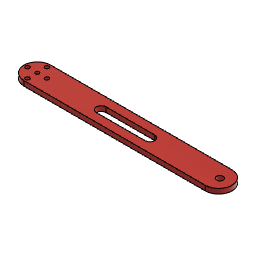
pendulum (Autodesk Fusion 360 design; units mm, degrees)
Autodesk Fusion 360 part; units mm, degrees
sketch "Sketch1" plane through (0, 0, 0) normal (0, 1, 0) x (1, 0, 0)
  line L0 (-90.5, 11) -> (80.5, 11)
  line L1 (80.5, 11) -> (80.5, -11)
  line L2 (80.5, -11) -> (-90.5, -11)
  line L3 (-90.5, -11) -> (-90.5, 11)
  circle A0 centre (-71.5, 0) radius 1.65
  circle A1 centre (-79.5, 8) radius 1.65
  circle A2 centre (-87.5, 0) radius 1.65
  circle A3 centre (-79.5, -8) radius 1.65
  circle A4 centre (70.5, 0) radius 2.75
  point P0 (-79.5, 0)
  dimension "d6" = 11
  dimension "d7" = 22
  dimension "d10" = 3.3
  dimension "d11" = 8
  dimension "d13" = 360
  dimension "d14" = 5.5
  dimension "d15" = 10
  dimension "d16" = 150
  dimension "d17" = 11
  dimension "d18" = 11
  dimension "d19" = 11
  constraint horizontal L0
  constraint vertical L1
  constraint horizontal L2
  constraint vertical L3
  measures "d6" distance of origin L2
  measures "d7" distance of L0.start L2.end
  measures "d10" diameter of A0
  measures "d11" distance of P0 A0.centre
  measures "d14" diameter of A4
  measures "d15" distance of L1 A4.centre
  measures "d16" distance of P0 A4.centre
  measures "d17" distance of L0 A4.centre
  measures "d18" distance of L0 P0
  measures "d19" distance of L3 P0
extrude "Extrude1" add sketch "Sketch1" along normal blind 4
fillet "Fillet1" radius 11 2 edges at (80.5, 2, -11) (80.5, 2, 11)
fillet "Fillet2" radius 11 2 edges at (-90.5, 2, 11) (-90.5, 2, -11)
sketch "Sketch3" plane through (0, 4, 0) normal (0, 1, 0) x (-1, 0, 0)
  circle A0 centre (79.5, -8) radius 1.65
  circle A1 centre (87.5, 0) radius 1.65
  circle A2 centre (79.5, 8) radius 1.65
  circle A3 centre (-70.5, 0) radius 2.75
  circle A4 centre (71.5, 0) radius 1.65
  arc A5 (79.5, -11) -> (79.5, 11) centre (79.5, 0) ccw
  line L0 (79.5, 11) -> (-69.5, 11)
  arc A6 (-69.5, 11) -> (-69.5, -11) centre (-69.5, 0) ccw
  line L1 (-69.5, -11) -> (79.5, -11)
  line L2 (27, 4) -> (-13, 4)
  arc A7 (-13, 4) -> (-13, -4) centre (-13, 0) ccw
  line L3 (-13, -4) -> (27, -4)
  arc A8 (27, -4) -> (27, 4) centre (27, 0) ccw
  line L4 (27, 0) -> (-13, 0) construction
  dimension "d24" = 8
  dimension "d30" = 40
  constraint tangent L2 A7
  constraint tangent A7 L3
  constraint parallel L2 L3
  constraint tangent L3 A8
  constraint tangent L2 A8
  constraint parallel L1 L4
  measures "d24" diameter of A7
  measures "d30" distance of A8.centre A7.centre
extrude "Extrude2" cut sketch "Sketch3" against normal up to surface (4 mm away) contours L2 A7 L3 A8
sketch "Sketch4" plane through (0, 4, 0) normal (0, 1, 0) x (-1, 0, 0)
  line L0 (27, -4) -> (-13, -4)
  arc A0 (-13, 4) -> (-13, -4) centre (-13, 0) ccw
  line L1 (-13, 4) -> (27, 4)
  arc A1 (27, -4) -> (27, 4) centre (27, 0) ccw
  circle A2 centre (79.5, -8) radius 1.65
  circle A3 centre (87.5, 0) radius 1.65
  circle A4 centre (79.5, 8) radius 1.65
  circle A5 centre (-70.5, 0) radius 2.75
  circle A6 centre (71.5, 0) radius 1.65
  arc A7 (79.5, -11) -> (79.5, 11) centre (79.5, 0) ccw
  line L2 (79.5, 11) -> (-69.5, 11)
  arc A8 (-69.5, 11) -> (-69.5, -11) centre (-69.5, 0) ccw
  line L3 (-69.5, -11) -> (79.5, -11)
  circle A9 centre (79.5, 0) radius 1.5
  dimension "d27" = 3
  constraint concentric A7 A9
  measures "d27" diameter of A9
extrude "Extrude3" cut sketch "Sketch4" against normal up to surface (4 mm away) contours A9
equation "length = 150 mm"
equation "width = 22 mm"
equation "thickness = 4 mm"
equation "d5 = length + width / 2"
equation "d6 = width / 2"
equation "d7 = width"
equation "d16 = length"
equation "d17 = width / 2"
equation "d18 = width / 2"
equation "d20 = thickness"
equation "d22 = width / 2"
equation "d23 = width / 2"
